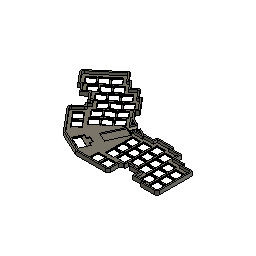
flynn (Autodesk Fusion 360 design; units mm, degrees)
Autodesk Fusion 360 part; units mm, degrees
(part 1 of 3)
sketch "Sketch1" plane through (0, 0, 0) normal (0, 1, 0) x (1, 0, 0)
  line L0 (0, 0) -> (0, -8) construction
  line L1 (0, -8) -> (8, -8) construction
  line L2 (8, -8) -> (22, -8)
  line L3 (22, -8) -> (22, -22)
  line L4 (22, -22) -> (8, -22)
  line L5 (8, -22) -> (8, -8)
  line L6 (8, -39) -> (8, -25)
  line L7 (8, -25) -> (22, -25)
  line L8 (22, -25) -> (22, -39)
  line L9 (22, -39) -> (8, -39)
  line L10 (8, -56) -> (8, -42)
  line L11 (8, -42) -> (22, -42)
  line L12 (22, -42) -> (22, -56)
  line L13 (22, -56) -> (8, -56)
  line L14 (22, -8) -> (22, -6) construction
  line L15 (22, -6) -> (26, -6) construction
  line L16 (26, -6) -> (40, -6)
  line L17 (40, -6) -> (40, -20)
  line L18 (40, -20) -> (26, -20)
  line L19 (26, -20) -> (26, -6)
  line L20 (26, -23) -> (40, -23)
  line L21 (40, -23) -> (40, -37)
  line L22 (40, -37) -> (26, -37)
  line L23 (26, -37) -> (26, -23)
  line L24 (26, -40) -> (40, -40)
  line L25 (40, -40) -> (40, -54)
  line L26 (40, -54) -> (26, -54)
  line L27 (26, -54) -> (26, -40)
  line L28 (40, -6) -> (40, 0) construction
  line L29 (40, 0) -> (44, 0) construction
  line L30 (44, 0) -> (58, 0)
  line L31 (58, 0) -> (58, -14)
  line L32 (58, -14) -> (44, -14)
  line L33 (44, -14) -> (44, 0)
  line L34 (58, -17) -> (58, -31)
  line L35 (44, -31) -> (44, -17)
  line L36 (58, -31) -> (44, -31)
  line L37 (44, -17) -> (58, -17)
  line L38 (58, -34) -> (58, -48)
  line L39 (44, -48) -> (44, -34)
  line L40 (58, -48) -> (44, -48)
  line L41 (44, -34) -> (58, -34)
  line L42 (58, 0) -> (62, 0) construction
  line L43 (62, 0) -> (62, -4) construction
  line L44 (62, -4) -> (76, -4)
  line L45 (76, -4) -> (76, -18)
  line L46 (76, -18) -> (62, -18)
  line L47 (62, -18) -> (62, -4)
  line L48 (76, -35) -> (62, -35)
  line L49 (62, -35) -> (62, -21)
  line L50 (76, -21) -> (76, -35)
  line L51 (62, -21) -> (76, -21)
  line L52 (76, -52) -> (62, -52)
  line L53 (62, -52) -> (62, -38)
  line L54 (76, -38) -> (76, -52)
  line L55 (62, -38) -> (76, -38)
  line L56 (76, -4) -> (80, -4) construction
  line L57 (80, -4) -> (80, -16) construction
  line L58 (80, -16) -> (94, -16)
  line L59 (94, -16) -> (94, -30)
  line L60 (94, -30) -> (80, -30)
  line L61 (80, -30) -> (80, -16)
  line L62 (94, -33) -> (94, -47)
  line L63 (80, -47) -> (80, -33)
  line L64 (94, -47) -> (80, -47)
  line L65 (80, -33) -> (94, -33)
  line L66 (94, -50) -> (94, -64)
  line L67 (80, -64) -> (80, -50)
  line L68 (94, -64) -> (80, -64)
  line L69 (80, -50) -> (94, -50)
  line L70 (94, -16) -> (98, -16) construction
  line L71 (98, -16) -> (98, -20) construction
  line L72 (98, -20) -> (112, -20)
  line L73 (112, -20) -> (112, -34)
  line L74 (112, -34) -> (98, -34)
  line L75 (98, -34) -> (98, -20)
  line L76 (98, -51) -> (98, -37)
  line L77 (112, -51) -> (98, -51)
  line L78 (112, -37) -> (112, -51)
  line L79 (98, -37) -> (112, -37)
  line L80 (98, -33) -> (98, -37) construction
  line L81 (98, -68) -> (98, -54)
  line L82 (112, -68) -> (98, -68)
  line L83 (112, -54) -> (112, -68)
  line L84 (98, -54) -> (112, -54)
  line L85 (98, -50) -> (98, -54) construction
  line L86 (22, -56) -> (22, -63) construction
  line L87 (22, -63) -> (19, -63) construction
  line L88 (19, -63) -> (33, -63)
  line L89 (33, -63) -> (33, -77)
  line L90 (33, -77) -> (19, -77)
  line L91 (19, -77) -> (19, -63)
  line L92 (15, -63) -> (15, -77)
  line L93 (1, -63) -> (15, -63)
  line L94 (4, -63) -> (1, -63) construction
  line L95 (15, -77) -> (1, -77)
  line L96 (1, -77) -> (1, -63)
  line L97 (26, -6) -> (26, 2) construction
  line L98 (26, 2) -> (18, 2) construction
  line L99 (40, 0) -> (48, 0) construction
  line L100 (44, 0) -> (44, 8) construction
  line L101 (44, 8) -> (36, 8) construction
  line L102 (58, 0) -> (58, 8) construction
  line L103 (58, 8) -> (66, 8) construction
  line L104 (62, -4) -> (62, 4) construction
  line L105 (62, 4) -> (70, 4) construction
  line L106 (76, -4) -> (76, 4) construction
  line L107 (76, 4) -> (84, 4) construction
  line L108 (80, -16) -> (80, -8) construction
  line L109 (80, -8) -> (88, -8) construction
  line L110 (94, -16) -> (94, -8) construction
  line L111 (94, -8) -> (102, -8) construction
  line L112 (98, -20) -> (98, -12) construction
  line L113 (98, -12) -> (106, -12) construction
  line L114 (112, -20) -> (112, -12) construction
  line L115 (112, -12) -> (120, -12) construction
  line L116 (0, 0) -> (18, 0)
  line L117 (18, 0) -> (18, 2)
  line L118 (18, 2) -> (36, 2)
  line L119 (36, 2) -> (36, 8)
  line L120 (36, 8) -> (61.9126, 8)
  line L121 (66, 8) -> (66, 4)
  line L122 (66, 4) -> (84, 4)
  line L123 (84, 4) -> (84, -8)
  line L124 (84, -8) -> (102, -8)
  line L125 (102, -8) -> (102, -12)
  line L126 (102, -12) -> (120, -12)
  line L127 (112, -68) -> (120, -68) construction
  line L128 (120, -68) -> (120, -76) construction
  line L129 (98, -68) -> (98, -76) construction
  line L130 (98, -76) -> (90, -76) construction
  line L131 (80, -64) -> (80, -72) construction
  line L132 (80, -72) -> (72, -72) construction
  line L133 (62, -52) -> (62, -60) construction
  line L134 (62, -60) -> (54, -60) construction
  line L135 (44, -48) -> (44, -56) construction
  line L136 (44, -56) -> (52, -56) construction
  line L137 (40, -54) -> (40, -62) construction
  line L138 (40, -62) -> (48, -62) construction
  line L139 (33, -63) -> (33, -55) construction
  line L140 (33, -55) -> (41, -55) construction
  line L141 (33, -77) -> (33, -85) construction
  line L142 (33, -85) -> (41, -85) construction
  line L143 (1, -77) -> (1, -85) construction
  line L144 (1, -85) -> (-7, -85) construction
  line L145 (1, -63) -> (1, -55) construction
  line L146 (1, -55) -> (-7, -55) construction
  line L147 (8, -56) -> (0, -56) construction
  line L148 (0, -56) -> (0, -48) construction
  line L149 (120, -12) -> (120, -76)
  line L150 (120, -76) -> (90, -76)
  line L151 (90, -76) -> (90, -72)
  line L152 (90, -72) -> (72, -72)
  line L153 (72, -72) -> (72, -60)
  line L154 (72, -60) -> (54, -60)
  line L155 (54, -60) -> (54, -56)
  line L156 (54, -56) -> (48, -56)
  line L157 (48, -56) -> (48, -62)
  line L158 (48, -62) -> (41, -62)
  line L159 (41, -62) -> (41, -85)
  line L160 (41, -85) -> (-7, -85)
  line L161 (-7, -85) -> (-7, -55)
  line L162 (-7, -55) -> (0, -55)
  line L163 (0, -55) -> (0, 0)
  line L164 (0, 0) -> (-4.5315, 2.1131)
  line L165 (-2.2658, 1.0565) -> (-5.5149, -5.9112)
  line L166 (-119.6157, 33.4759) -> (-108.8911, 42.4749)
  line L167 (-48.5486, -6.1026) -> (-39.5496, -16.8273)
  line L168 (-84.729, -22.1021) -> (-75.7299, -32.8267)
  line L169 (-14.5696, 17.1875) -> (-26.1398, 30.9763)
  line L170 (-65.0053, -23.8277) -> (-74.0043, -13.1031)
  line L171 (-19.7119, 23.3158) -> (-14.5696, 17.1875) construction
  line L172 (-95.9996, -21.116) -> (-65.1458, -57.8862)
  line L173 (-117.5376, 24.7764) -> (-105.9674, 10.9876)
  line L174 (-62.4342, -26.8919) -> (-73.1588, -35.8909)
  line L175 (-139.8854, 45.1866) -> (-120.6018, 22.2052)
  line L176 (-23.2691, 15.1093) -> (-25.8403, 18.1735) construction
  line L177 (-128.6148, 44.2005) -> (-133.7571, 50.3289) construction
  line L178 (-37.824, 2.8964) -> (-48.5486, -6.1026)
  line L179 (-82.4931, 35.9065) -> (-93.2177, 26.9075)
  line L180 (-105.9674, 10.9876) -> (-96.7749, 18.701)
  line L181 (-53.4351, -37.6165) -> (-62.4342, -26.8919)
  line L182 (-100.9577, 43.9103) -> (-91.9586, 33.1856)
  line L183 (-56.5616, 15.8926) -> (-45.8369, 24.8917)
  line L184 (-46.664, -33.2402) -> (-4.5315, 2.1131)
  line L185 (-55.3635, -35.3184) -> (-53.4351, -37.6165) construction
  line L186 (-71.1959, 27.1103) -> (-60.4713, 36.1093)
  line L187 (-125.7441, 28.3336) -> (-120.6018, 22.2052) construction
  line L188 (-69.4703, 46.8339) -> (-80.195, 37.8349)
  line L189 (-61.5714, -17.03) -> (-52.5723, -27.7547)
  line L190 (-108.8911, 42.4749) -> (-117.8902, 53.1995)
  line L191 (-104.9814, 22.2582) -> (-111.1097, 17.1159) construction
  line L192 (-91.8446, 75.0543) -> (-102.5693, 66.0553)
  line L193 (-77.2103, 63.8367) -> (-87.9349, 54.8376)
  line L194 (-47.43, -33.883) -> (-41.3017, -28.7407) construction
  line L195 (-93.5702, 55.3307) -> (-82.8456, 64.3297)
  line L196 (-50.8467, -8.031) -> (-61.5714, -17.03)
  line L197 (-94.2568, 31.2573) -> (-103.2558, 41.9819)
  line L198 (-64.1597, -46.6155) -> (-53.4351, -37.6165)
  line L199 (-42.1645, -38.6025) -> (-46.664, -33.2402)
  line L200 (-120.6018, 22.2052) -> (-117.5376, 24.7764)
  line L201 (-70.2881, -51.7578) -> (-65.1458, -57.8862) construction
  line L202 (-4.5315, 2.1131) -> (0, 0)
  line L203 (-102.5693, 66.0553) -> (-93.5702, 55.3307)
  line L204 (-55.4615, 69.032) -> (-64.6541, 61.3185)
  line L205 (-75.7299, -32.8267) -> (-65.0053, -23.8277)
  line L206 (-16.1017, 15.9019) -> (-14.5696, 17.1875)
  line L207 (-113.9804, 32.9829) -> (-104.9814, 22.2582)
  line L208 (-26.1398, 30.9763) -> (-21.5435, 34.833)
  line L209 (-24.8012, 13.8238) -> (-35.5258, 4.8247)
  line L210 (-115.592, 55.1279) -> (-106.593, 44.4033)
  line L211 (-76.7173, 69.472) -> (-81.8596, 75.6004) construction
  line L212 (-111.1097, 17.1159) -> (-105.9674, 10.9876) construction
  line L213 (-87.9349, 54.8376) -> (-78.9359, 44.113)
  line L214 (-56.4476, 57.7613) -> (-50.3192, 62.9036) construction
  line L215 (-56.4476, 57.7613) -> (-59.0187, 60.8255) construction
  line L216 (-74.0043, -13.1031) -> (-67.876, -7.9608) construction
  line L217 (-82.8456, 64.3297) -> (-76.7173, 69.472) construction
  line L218 (-56.4476, 57.7613) -> (-67.1722, 48.7623)
  line L219 (-76.2242, 75.1073) -> (-79.2884, 72.5362)
  line L220 (-91.9586, 33.1856) -> (-81.234, 42.1847)
  line L221 (-32.8142, 35.819) -> (-41.8132, 46.5437)
  line L222 (-81.234, 42.1847) -> (-90.233, 52.9093)
  line L223 (-25.8403, 18.1735) -> (-19.7119, 23.3158) construction
  line L224 (-61.5714, -17.03) -> (-66.9337, -21.5296) construction
  line L225 (-74.0043, -13.1031) -> (-84.729, -22.1021)
  line L226 (-90.233, 52.9093) -> (-100.9577, 43.9103)
  line L227 (-69.5843, 4.9652) -> (-75.7127, -0.1771) construction
  line L228 (-47.3068, -32.4742) -> (-42.1645, -38.6025) construction
  line L229 (-47.4485, 47.0367) -> (-41.3202, 52.179) construction
  line L230 (-59.0187, 60.8255) -> (-68.2113, 53.112) construction
  line L231 (-77.2103, 63.8367) -> (-79.7814, 66.9008) construction
  line L232 (-4.5315, 2.1131) -> (-10.6599, -3.0292) construction
  line L233 (-84.2187, 16.1829) -> (-73.4941, 25.1819)
  line L234 (-65.5606, 26.6173) -> (-56.5616, 15.8926)
  line L235 (-10.6599, -3.0292) -> (-15.8022, 3.0991) construction
  line L236 (-28.825, -7.8282) -> (-37.824, 2.8964)
  line L237 (-77.7378, -7.098) -> (-82.8801, -0.9696) construction
  line L238 (-49.5877, -1.7529) -> (-38.863, 7.2461)
  line L239 (-52.5723, -27.7547) -> (-41.8477, -18.7556)
  line L240 (-58.1732, 38.0377) -> (-47.4485, 47.0367)
  line L241 (-58.8597, 13.9643) -> (-67.8587, 24.6889)
  line L242 (-68.2113, 53.112) -> (-62.0829, 58.2543) construction
  line L243 (-92.8042, 55.9735) -> (-95.8684, 53.4023) construction
  line L244 (-43.8913, 55.2432) -> (-55.4615, 69.032)
  line L245 (-2.2658, 1.0565) -> (-5.5149, -5.9112)
  line L246 (-47.4485, 47.0367) -> (-56.4476, 57.7613)
  line L247 (-67.1722, 48.7623) -> (-58.1732, 38.0377)
  line L248 (-60.4713, 36.1093) -> (-69.4703, 46.8339)
  line L249 (-15.8022, 3.0991) -> (-24.8012, 13.8238)
  line L250 (-96.7749, 18.701) -> (-85.2047, 4.9122)
  line L251 (-85.7163, 80.1966) -> (-90.8586, 86.325) construction
  line L252 (-117.8902, 53.1995) -> (-128.6148, 44.2005)
  line L253 (-71.6094, -1.9557) -> (-77.7378, -7.098) construction
  line L254 (-105.8269, 45.0461) -> (-108.8911, 42.4749) construction
  line L255 (-60.8848, 7.0434) -> (-71.6094, -1.9557)
  line L256 (-84.729, -22.1021) -> (-90.8573, -27.2444) construction
  line L257 (-79.7814, 66.9008) -> (-82.8456, 64.3297) construction
  line L258 (-34.8393, 28.8981) -> (-30.243, 32.7549) construction
  line L259 (-78.2838, 2.8871) -> (-82.8801, -0.9696)
  line L260 (-79.2884, 72.5362) -> (-90.8586, 86.325)
  line L261 (-62.6104, -12.6803) -> (-51.8858, -3.6813)
  line L262 (-34.8393, 28.8981) -> (-45.5639, 19.8991)
  line L263 (-41.8132, 46.5437) -> (-44.3844, 49.6078) construction
  line L264 (-85.2047, 4.9122) -> (-82.1406, 7.4834)
  line L265 (-41.3202, 52.179) -> (-46.4625, 58.3074) construction
  line L266 (-64.6541, 61.3185) -> (-76.2242, 75.1073)
  line L267 (-69.5843, 4.9652) -> (-58.8597, 13.9643)
  line L268 (-82.8801, -0.9696) -> (-78.3806, -6.3319)
  line L269 (-47.8621, 17.9708) -> (-58.5867, 8.9717)
  line L270 (-30.243, 32.7549) -> (-35.3853, 38.8832) construction
  line L271 (-41.8132, 46.5437) -> (-52.5378, 37.5446)
  line L272 (-45.8369, 24.8917) -> (-54.836, 35.6163)
  line L273 (-35.6849, 51.686) -> (-40.8272, 57.8143) construction
  line L274 (-82.8456, 64.3297) -> (-91.8446, 75.0543)
  line L275 (-78.3806, -6.3319) -> (-95.9996, -21.116)
  line L276 (-58.5867, 8.9717) -> (-49.5877, -1.7529)
  line L277 (-71.6094, -1.9557) -> (-62.6104, -12.6803)
  line L278 (-77.2103, 63.8367) -> (-71.0819, 68.979) construction
  line L279 (-67.876, -7.9608) -> (-73.0183, -1.8324) construction
  line L280 (-32.8142, 35.819) -> (-26.6858, 40.9613) construction
  line L281 (-41.8132, 46.5437) -> (-35.6849, 51.686) construction
  line L282 (-40.8272, 57.8143) -> (-43.8913, 55.2432)
  line L283 (-91.8446, 75.0543) -> (-85.7163, 80.1966) construction
  line L284 (-75.7127, -0.1771) -> (-80.855, 5.9513) construction
  line L285 (-50.3192, 62.9036) -> (-55.4615, 69.032) construction
  line L286 (-78.5834, 15.6899) -> (-69.5843, 4.9652)
  line L287 (-84.2187, 16.1829) -> (-90.347, 11.0406) construction
  line L288 (-90.347, 11.0406) -> (-85.2047, 4.9122) construction
  line L289 (-45.5639, 19.8991) -> (-36.5649, 9.1745)
  line L290 (-43.5388, 26.82) -> (-32.8142, 35.819)
  line L291 (-38.863, 7.2461) -> (-47.8621, 17.9708)
  line L292 (-25.8403, 18.1735) -> (-34.8393, 28.8981)
  line L293 (-51.8858, -3.6813) -> (-60.8848, 7.0434)
  line L294 (-90.8573, -27.2444) -> (-95.9996, -21.116) construction
  line L295 (-82.1406, 7.4834) -> (-78.2838, 2.8871)
  line L296 (-26.6858, 40.9613) -> (-21.5435, 34.833) construction
  line L297 (-68.2113, 53.112) -> (-77.2103, 63.8367)
  line L298 (-71.0819, 68.979) -> (-76.2242, 75.1073) construction
  line L299 (-21.5435, 34.833) -> (-38.1998, 54.6832)
  line L300 (-67.8587, 24.6889) -> (-78.5834, 15.6899)
  line L301 (-30.243, 32.7549) -> (-32.8142, 35.819) construction
  line L302 (-44.3844, 49.6078) -> (-47.4485, 47.0367) construction
  line L303 (-52.5378, 37.5446) -> (-43.5388, 26.82)
  line L304 (-62.0829, 58.2543) -> (-67.2252, 64.3827) construction
  line L305 (-36.5649, 9.1745) -> (-25.8403, 18.1735)
  line L306 (-128.6148, 44.2005) -> (-119.6157, 33.4759)
  line L307 (-54.836, 35.6163) -> (-65.5606, 26.6173)
  line L308 (-104.9814, 22.2582) -> (-94.2568, 31.2573)
  line L309 (-90.8586, 86.325) -> (-139.8854, 45.1866)
  line L310 (-106.593, 44.4033) -> (-95.8684, 53.4023)
  line L311 (-52.5723, -27.7547) -> (-47.43, -33.883) construction
  line L312 (-95.8684, 53.4023) -> (-104.8674, 64.1269)
  line L313 (-39.5496, -16.8273) -> (-28.825, -7.8282)
  line L314 (-66.9337, -21.5296) -> (-65.0053, -23.8277) construction
  line L315 (-53.4351, -37.6165) -> (-47.3068, -32.4742) construction
  line L316 (-133.7571, 50.3289) -> (-139.8854, 45.1866) construction
  line L317 (-78.9359, 44.113) -> (-68.2113, 53.112)
  line L318 (-64.1597, -46.6155) -> (-70.2881, -51.7578) construction
  line L319 (-80.195, 37.8349) -> (-71.1959, 27.1103)
  line L320 (-4.5315, 2.1131) -> (-16.1017, 15.9019)
  line L321 (-65.1458, -57.8862) -> (-42.1645, -38.6025)
  line L322 (-103.2558, 41.9819) -> (-113.9804, 32.9829)
  line L323 (-73.1588, -35.8909) -> (-64.1597, -46.6155)
  line L324 (-93.2177, 26.9075) -> (-84.2187, 16.1829)
  line L325 (-73.4941, 25.1819) -> (-82.4931, 35.9065)
  line L326 (-41.8477, -18.7556) -> (-50.8467, -8.031)
  line L327 (-24.8012, 13.8238) -> (-23.2691, 15.1093) construction
  line L328 (-104.8674, 64.1269) -> (-115.592, 55.1279)
  line L329 (-119.6157, 33.4759) -> (-125.7441, 28.3336) construction
  line L330 (-26.5268, -5.8999) -> (-15.8022, 3.0991)
  line L331 (-35.5258, 4.8247) -> (-26.5268, -5.8999)
  line L332 (-7, -85) -> (-17, -85)
  line L333 (-65.1458, -57.8862) -> (-58.7179, -65.5466)
  line L334 (-58.7179, -65.5466) -> (-17, -85)
  line L335 (61.9126, 8) -> (66, 8)
  line L336 (-40.8272, 57.8143) -> (-35.6849, 51.686)
  point P0 (-4.5315, 2.1131)
  dimension "d1" = 8
  dimension "d3" = 14
  dimension "d4" = 14
  dimension "d7" = 0
  dimension "d8" = -17
  dimension "d9" = 2
  dimension "d10" = 4
  dimension "d11" = 14
  dimension "d12" = 14
  dimension "d15" = 0
  dimension "d16" = -17
  dimension "d17" = 14
  dimension "d18" = 14
  dimension "d19" = 4
  dimension "d20" = 6
  dimension "d23" = 0
  dimension "d24" = -17
  dimension "d25" = 4
  dimension "d26" = 4
  dimension "d27" = 14
  dimension "d28" = 14
  dimension "d31" = 0
  dimension "d32" = -17
  dimension "d33" = 12
  dimension "d34" = 4
  dimension "d35" = 14
  dimension "d36" = 14
  dimension "d39" = 0
  dimension "d40" = -17
  dimension "d41" = 4
  dimension "d42" = 4
  dimension "d43" = 14
  dimension "d44" = 14
  dimension "d47" = 0
  dimension "d48" = -17
  dimension "d49" = 14
  dimension "d50" = 14
  dimension "d51" = 7
  dimension "d52" = 3
  dimension "d55" = -18
  dimension "d56" = 0
  dimension "d57" = 5
  dimension "d58" = 155
  dimension "d68" = 10
  constraint coincident L0.start L116.start
  constraint vertical L0
  constraint perpendicular L0 L1
  constraint horizontal L2
  constraint vertical L3
  constraint horizontal L4
  constraint vertical L5
  constraint perpendicular L2 L14
  constraint perpendicular L14 L15
  constraint horizontal L16
  constraint vertical L17
  constraint horizontal L18
  constraint vertical L19
  constraint perpendicular L16 L28
  constraint perpendicular L28 L29
  constraint horizontal L30
  constraint vertical L31
  constraint horizontal L32
  constraint vertical L33
  constraint perpendicular L31 L42
  constraint perpendicular L30 L43
  constraint horizontal L44
  constraint vertical L45
  constraint horizontal L46
  constraint vertical L47
  constraint perpendicular L45 L56
  constraint perpendicular L56 L57
  constraint horizontal L58
  constraint vertical L59
  constraint horizontal L60
  constraint vertical L61
  constraint perpendicular L59 L70
  constraint perpendicular L58 L71
  constraint horizontal L72
  constraint vertical L73
  constraint horizontal L74
  constraint vertical L75
  constraint perpendicular L13 L86
  constraint perpendicular L86 L87
  constraint horizontal L88
  constraint vertical L89
  constraint horizontal L90
  constraint vertical L91
  constraint equal L0 L1
  constraint perpendicular L16 L97
  constraint perpendicular L19 L98
  constraint equal L0 L97
  constraint equal L0 L98
  constraint coincident L30 L99.end
  constraint equal L0 L99
  constraint perpendicular L99 L100
  constraint perpendicular L100 L101
  constraint equal L0 L100
  constraint equal L0 L101
  constraint perpendicular L30 L102
  constraint perpendicular L102 L103
  constraint equal L0 L102
  constraint equal L0 L103
  constraint perpendicular L44 L104
  constraint perpendicular L104 L105
  constraint equal L103 L105
  constraint equal L102 L104
  constraint perpendicular L56 L106
  constraint perpendicular L106 L107
  constraint equal L0 L107
  constraint equal L0 L106
  constraint coincident L57 L108.end
  constraint perpendicular L58 L108
  constraint perpendicular L108 L109
  constraint equal L0 L109
  constraint equal L0 L108
  constraint perpendicular L70 L110
  constraint perpendicular L59 L111
  constraint equal L0 L111
  constraint equal L0 L110
  constraint perpendicular L70 L112
  constraint perpendicular L112 L113
  constraint equal L0 L113
  constraint equal L0 L112
  constraint perpendicular L72 L114
  constraint perpendicular L114 L115
  constraint equal L0 L115
  constraint equal L0 L114
  constraint perpendicular L97 L116
  constraint perpendicular L98 L117
  constraint perpendicular L117 L118
  constraint perpendicular L101 L119
  constraint perpendicular L119 L120
  constraint coincident L105 L121.end
  constraint perpendicular L105 L121
  constraint coincident L109 L123.end
  constraint perpendicular L109 L123
  constraint coincident L113 L125.end
  constraint perpendicular L113 L125
  constraint perpendicular L83 L127
  constraint perpendicular L82 L128
  constraint equal L0 L127
  constraint equal L0 L128
  constraint perpendicular L82 L129
  constraint perpendicular L129 L130
  constraint equal L0 L129
  constraint equal L0 L130
  constraint perpendicular L68 L131
  constraint perpendicular L131 L132
  constraint equal L0 L131
  constraint equal L0 L132
  constraint perpendicular L52 L133
  constraint perpendicular L53 L134
  constraint equal L0 L133
  constraint equal L0 L134
  constraint perpendicular L40 L135
  constraint perpendicular L135 L136
  constraint equal L0 L135
  constraint equal L0 L136
  constraint perpendicular L26 L137
  constraint perpendicular L137 L138
  constraint equal L0 L137
  constraint equal L0 L138
  constraint perpendicular L88 L139
  constraint perpendicular L139 L140
  constraint equal L0 L140
  constraint equal L0 L139
  constraint perpendicular L90 L141
  constraint perpendicular L141 L142
  constraint equal L0 L141
  constraint equal L0 L142
  constraint perpendicular L95 L143
  constraint perpendicular L143 L144
  constraint equal L0 L143
  constraint equal L0 L144
  constraint perpendicular L93 L145
  constraint perpendicular L96 L146
  constraint equal L0 L145
  constraint equal L0 L146
  constraint perpendicular L10 L147
  constraint perpendicular L13 L148
  constraint equal L0 L148
  constraint equal L0 L147
  constraint perpendicular L132 L151
  constraint perpendicular L131 L152
  constraint perpendicular L134 L153
  constraint perpendicular L133 L154
  constraint perpendicular L136 L155
  constraint coincident L136 L156.end
  constraint perpendicular L155 L156
  constraint perpendicular L138 L157
  constraint perpendicular L137 L158
  constraint perpendicular L142 L159
  constraint perpendicular L148 L162
  constraint perpendicular L116 L163
  constraint midpoint L164 L165.start
  constraint perpendicular L164 L165
  constraint symmetric L0.start L165 L164.end
  constraint symmetric L0.start L165 P0
  constraint symmetric L0.end L165 L232.end
  constraint symmetric L1.end L165 L235.end
  constraint symmetric L2.end L165 L209.start
  constraint symmetric L3.end L165 L209.end
  constraint symmetric L4.end L165 L330.start
  constraint symmetric L6.start L165 L167.end
  constraint symmetric L6.end L165 L236.start
  constraint symmetric L7.end L165 L178.start
  constraint symmetric L8.end L165 L167.start
  constraint symmetric L10.start L165 L189.end
  constraint symmetric L10.end L165 L239.end
  constraint symmetric L11.end L165 L196.start
  constraint symmetric L12.end L165 L189.start
  constraint symmetric L14.end L165 L176.start
  constraint symmetric L15.end L165 L176.end
  constraint symmetric L16.end L165 L258.start
  constraint symmetric L17.end L165 L262.end
  constraint symmetric L18.end L165 L289.end
  constraint symmetric L21.end L165 L269.end
  constraint symmetric L20.start L165 L238.end
  constraint symmetric L20.end L165 L269.start
  constraint symmetric L22.end L165 L238.start
  constraint symmetric L25.end L165 L253.start
  constraint symmetric L24.start L165 L261.end
  constraint symmetric L24.end L165 L255.start
  constraint symmetric L26.end L165 L261.start
  constraint symmetric L28.end L165 L258.end
  constraint symmetric L29.end L165 L221.start
  constraint symmetric L30.end L165 L221.end
  constraint symmetric L31.end L165 L271.end
  constraint symmetric L32.end L165 L290.start
  constraint symmetric L34.start L165 L272.end
  constraint symmetric L34.end L165 L234.start
  constraint symmetric L35.start L165 L183.start
  constraint symmetric L35.end L165 L183.end
  constraint symmetric L38.start L165 L241.end
  constraint symmetric L38.end L165 L286.start
  constraint symmetric L39.start L165 L227.start
  constraint symmetric L39.end L165 L241.start
  constraint symmetric L42.end L165 L263.end
  constraint symmetric L43.end L165 L229.start
  constraint symmetric L44.end L165 L214.start
  constraint symmetric L45.end L165 L218.end
  constraint symmetric L46.end L165 L240.start
  constraint symmetric L48.start L165 L188.end
  constraint symmetric L48.end L165 L186.start
  constraint symmetric L49.end L165 L186.end
  constraint symmetric L50.start L165 L188.start
  constraint symmetric L52.start L165 L179.end
  constraint symmetric L52.end L165 L233.start
  constraint symmetric L53.end L165 L233.end
  constraint symmetric L54.start L165 L179.start
  constraint symmetric L56.end L165 L215.end
  constraint symmetric L57.end L165 L230.end
  constraint symmetric L58.end L165 L193.start
  constraint symmetric L59.end L165 L193.end
  constraint symmetric L60.end L165 L213.end
  constraint symmetric L63.end L165 L220.end
  constraint symmetric L62.start L165 L222.end
  constraint symmetric L62.end L165 L182.start
  constraint symmetric L63.start L165 L182.end
  constraint symmetric L67.end L165 L197.start
  constraint symmetric L66.start L165 L197.end
  constraint symmetric L66.end L165 L207.start
  constraint symmetric L67.start L165 L191.start
  constraint symmetric L70.end L165 L231.end
  constraint symmetric L71.end L165 L195.end
  constraint symmetric L72.end L165 L192.start
  constraint symmetric L73.end L165 L192.end
  constraint symmetric L74.end L165 L195.start
  constraint symmetric L76.start L165 L210.end
  constraint symmetric L76.end L165 L243.end
  constraint symmetric L77.start L165 L210.start
  constraint symmetric L78.start L165 L312.end
  constraint symmetric L80.start L165 L243.start
  constraint symmetric L81.start L165 L166.start
  constraint symmetric L81.end L165 L166.end
  constraint symmetric L82.start L165 L177.start
  constraint symmetric L83.start L165 L190.end
  constraint symmetric L85.start L165 L254.start
  constraint symmetric L86.end L165 L224.end
  constraint symmetric L87.end L165 L170.start
  constraint symmetric L88.end L165 L170.end
  constraint symmetric L89.end L165 L168.start
  constraint symmetric L90.end L165 L168.end
  constraint symmetric L95.end L165 L198.start
  constraint symmetric L92.start L165 L174.start
  constraint symmetric L92.end L165 L174.end
  constraint symmetric L93.start L165 L181.start
  constraint symmetric L94.start L165 L185.start
  constraint symmetric L97.end L165 L171.start
  constraint symmetric L98.end L165 L169.start
  constraint symmetric L99.end L165 L270.end
  constraint symmetric L100.end L165 L280.end
  constraint symmetric L101.end L165 L208.end
  constraint symmetric L102.end L165 L273.start
  constraint symmetric L103.end L165 L273.end
  constraint symmetric L104.end L165 L229.end
  constraint symmetric L105.end L165 L265.end
  constraint symmetric L106.end L165 L214.end
  constraint symmetric L107.end L165 L204.start
  constraint symmetric L108.end L165 L242.end
  constraint symmetric L109.end L165 L304.end
  constraint symmetric L110.end L165 L278.end
  constraint symmetric L111.end L165 L219.start
  constraint symmetric L112.end L165 L211.start
  constraint symmetric L113.end L165 L211.end
  constraint symmetric L114.end L165 L251.start
  constraint symmetric L115.end L165 L251.end
  constraint symmetric L116.end L165 L206.start
  constraint symmetric L118.end L165 L169.end
  constraint symmetric L120.end L165 L299.end
  constraint symmetric L121.end L165 L244.start
  constraint symmetric L123.end L165 L204.end
  constraint symmetric L125.end L165 L219.end
  constraint symmetric L127.end L165 L177.end
  constraint symmetric L128.end L165 L175.start
  constraint symmetric L129.end L165 L187.start
  constraint symmetric L130.end L165 L175.end
  constraint symmetric L131.end L165 L191.end
  constraint symmetric L132.end L165 L173.end
  constraint symmetric L133.end L165 L287.end
  constraint symmetric L134.end L165 L250.end
  constraint symmetric L135.end L165 L227.end
  constraint symmetric L136.end L165 L284.end
  constraint symmetric L137.end L165 L237.start
  constraint symmetric L138.end L165 L237.end
  constraint symmetric L139.end L165 L216.end
  constraint symmetric L140.end L165 L279.end
  constraint symmetric L141.end L165 L256.end
  constraint symmetric L142.end L165 L172.start
  constraint symmetric L143.end L165 L201.start
  constraint symmetric L144.end L165 L172.end
  constraint symmetric L145.end L165 L228.start
  constraint symmetric L146.end L165 L199.start
  constraint symmetric L147.end L165 L194.start
  constraint symmetric L148.end L165 L194.end
  constraint symmetric L151.end L165 L173.start
  constraint symmetric L153.end L165 L180.end
  constraint symmetric L155.end L165 L264.end
  constraint symmetric L156.end L165 L259.start
  constraint symmetric L158.end L165 L268.end
  constraint symmetric L162.end L165 L184.start
  constraint symmetric P0 L165 L0.start
  constraint symmetric L245.start L165 L165.start
  constraint symmetric L245.end L165 L165.end
  constraint perpendicular L161 L332
  constraint perpendicular L321 L333
  constraint equal L332 L333
  constraint perpendicular L121 L335
  measures "d1" distance of L0.start L0.end
  measures "d3" distance of L1.end L2.end
  measures "d4" distance of L1.end L4.end
  measures "d9" distance of L2.end L14.end
  measures "d10" distance of L14.end L15.end
  measures "d11" distance of L15.end L16.end
  measures "d12" distance of L15.end L18.end
  measures "d17" distance of L29.end L30.end
  measures "d18" distance of L29.end L32.end
  measures "d19" distance of L28.end L29.end
  measures "d20" distance of L16.end L28.end
  measures "d25" distance of L30.end L42.end
  measures "d26" distance of L42.end L43.end
  measures "d27" distance of L43.end L44.end
  measures "d28" distance of L43.end L46.end
  measures "d33" distance of L56.end L57.end
  measures "d34" distance of L44.end L56.end
  measures "d35" distance of L57.end L58.end
  measures "d36" distance of L57.end L60.end
  measures "d41" distance of L58.end L70.end
  measures "d42" distance of L70.end L71.end
  measures "d43" distance of L71.end L72.end
  measures "d44" distance of L71.end L74.end
  measures "d49" distance of L87.end L88.end
  measures "d50" distance of L87.end L90.end
  measures "d51" distance of L12.end L86.end
  measures "d52" distance of L86.end L87.end
  measures "d57" distance of L0.start P0
  measures "d58" angle of L116 L164
  measures "d68" distance of L172.end L333.end
extrude "Extrude1" add sketch "Sketch1" along normal blind 1.3
sketch "Sketch15" plane through (0, 1.3, 0) normal (0, 1, 0) x (-1, 0, 0)
  line L0 (91.8446, -75.0543) -> (82.8456, -64.3297)
  line L1 (82.8456, -64.3297) -> (93.5702, -55.3307)
  line L2 (93.5702, -55.3307) -> (102.5693, -66.0553)
  line L3 (102.5693, -66.0553) -> (91.8446, -75.0543)
  line L4 (100.9577, -43.9103) -> (90.233, -52.9093)
  line L5 (90.233, -52.9093) -> (81.234, -42.1847)
  line L6 (81.234, -42.1847) -> (91.9586, -33.1856)
  line L7 (91.9586, -33.1856) -> (100.9577, -43.9103)
  line L8 (58.1732, -38.0377) -> (67.1722, -48.7623)
  line L9 (67.1722, -48.7623) -> (56.4476, -57.7613)
  line L10 (56.4476, -57.7613) -> (47.4485, -47.0367)
  line L11 (47.4485, -47.0367) -> (58.1732, -38.0377)
  line L12 (43.5388, -26.82) -> (52.5378, -37.5446)
  line L13 (52.5378, -37.5446) -> (41.8132, -46.5437)
  line L14 (41.8132, -46.5437) -> (32.8142, -35.819)
  line L15 (32.8142, -35.819) -> (43.5388, -26.82)
  line L16 (78.5834, -15.6899) -> (67.8587, -24.6889)
  line L17 (67.8587, -24.6889) -> (58.8597, -13.9643)
  line L18 (58.8597, -13.9643) -> (69.5843, -4.9652)
  line L19 (69.5843, -4.9652) -> (78.5834, -15.6899)
  line L20 (60.8848, -7.0434) -> (51.8858, 3.6813)
  line L21 (51.8858, 3.6813) -> (62.6104, 12.6803)
  line L22 (62.6104, 12.6803) -> (71.6094, 1.9557)
  line L23 (71.6094, 1.9557) -> (60.8848, -7.0434)
  line L24 (47.8621, -17.9708) -> (38.863, -7.2461)
  line L25 (38.863, -7.2461) -> (49.5877, 1.7529)
  line L26 (49.5877, 1.7529) -> (58.5867, -8.9717)
  line L27 (58.5867, -8.9717) -> (47.8621, -17.9708)
  line L28 (25.8403, -18.1735) -> (36.5649, -9.1745)
  line L29 (36.5649, -9.1745) -> (45.5639, -19.8991)
  line L30 (45.5639, -19.8991) -> (34.8393, -28.8981)
  line L31 (34.8393, -28.8981) -> (25.8403, -18.1735)
  line L32 (119.6157, -33.4759) -> (128.6148, -44.2005)
  line L33 (128.6148, -44.2005) -> (117.8902, -53.1995)
  line L34 (117.8902, -53.1995) -> (108.8911, -42.4749)
  line L35 (108.8911, -42.4749) -> (119.6157, -33.4759)
  line L36 (65.5606, -26.6173) -> (54.836, -35.6163)
  line L37 (54.836, -35.6163) -> (45.8369, -24.8917)
  line L38 (45.8369, -24.8917) -> (56.5616, -15.8926)
  line L39 (56.5616, -15.8926) -> (65.5606, -26.6173)
  line L40 (28.825, 7.8282) -> (39.5496, 16.8273)
  line L41 (39.5496, 16.8273) -> (48.5486, 6.1026)
  line L42 (48.5486, 6.1026) -> (37.824, -2.8964)
  line L43 (37.824, -2.8964) -> (28.825, 7.8282)
  line L44 (68.2113, -53.112) -> (78.9359, -44.113)
  line L45 (78.9359, -44.113) -> (87.9349, -54.8376)
  line L46 (87.9349, -54.8376) -> (77.2103, -63.8367)
  line L47 (77.2103, -63.8367) -> (68.2113, -53.112)
  line L48 (71.1959, -27.1103) -> (80.195, -37.8349)
  line L49 (80.195, -37.8349) -> (69.4703, -46.8339)
  line L50 (69.4703, -46.8339) -> (60.4713, -36.1093)
  line L51 (60.4713, -36.1093) -> (71.1959, -27.1103)
  line L52 (113.9804, -32.9829) -> (103.2558, -41.9819)
  line L53 (103.2558, -41.9819) -> (94.2568, -31.2573)
  line L54 (94.2568, -31.2573) -> (104.9814, -22.2582)
  line L55 (104.9814, -22.2582) -> (113.9804, -32.9829)
  line L56 (64.1597, 46.6155) -> (73.1588, 35.8909)
  line L57 (73.1588, 35.8909) -> (62.4342, 26.8919)
  line L58 (62.4342, 26.8919) -> (53.4351, 37.6165)
  line L59 (53.4351, 37.6165) -> (64.1597, 46.6155)
  line L60 (82.4931, -35.9065) -> (73.4941, -25.1819)
  line L61 (73.4941, -25.1819) -> (84.2187, -16.1829)
  line L62 (84.2187, -16.1829) -> (93.2177, -26.9075)
  line L63 (93.2177, -26.9075) -> (82.4931, -35.9065)
  line L64 (50.8467, 8.031) -> (41.8477, 18.7556)
  line L65 (41.8477, 18.7556) -> (52.5723, 27.7547)
  line L66 (52.5723, 27.7547) -> (61.5714, 17.03)
  line L67 (61.5714, 17.03) -> (50.8467, 8.031)
  line L68 (115.592, -55.1279) -> (104.8674, -64.1269)
  line L69 (104.8674, -64.1269) -> (95.8684, -53.4023)
  line L70 (95.8684, -53.4023) -> (106.593, -44.4033)
  line L71 (106.593, -44.4033) -> (115.592, -55.1279)
  line L72 (-15, 77) -> (-1, 77)
  line L73 (-1, 77) -> (-1, 63)
  line L74 (-1, 63) -> (-15, 63)
  line L75 (-15, 63) -> (-15, 77)
  line L76 (84.729, 22.1021) -> (74.0043, 13.1031)
  line L77 (74.0043, 13.1031) -> (65.0053, 23.8277)
  line L78 (65.0053, 23.8277) -> (75.7299, 32.8267)
  line L79 (75.7299, 32.8267) -> (84.729, 22.1021)
  line L80 (-33, 77) -> (-19, 77)
  line L81 (-19, 77) -> (-19, 63)
  line L82 (-19, 63) -> (-33, 63)
  line L83 (-33, 63) -> (-33, 77)
  line L84 (-98, 68) -> (-98, 54)
  line L85 (-98, 54) -> (-112, 54)
  line L86 (-112, 54) -> (-112, 68)
  line L87 (-112, 68) -> (-98, 68)
  line L88 (-98, 51) -> (-98, 37)
  line L89 (-98, 37) -> (-112, 37)
  line L90 (-112, 37) -> (-112, 51)
  line L91 (-112, 51) -> (-98, 51)
  line L92 (-62, 52) -> (-62, 38)
  line L93 (-62, 38) -> (-76, 38)
  line L94 (-76, 38) -> (-76, 52)
  line L95 (-76, 52) -> (-62, 52)
  line L96 (-112, 34) -> (-98, 34)
  line L97 (-98, 34) -> (-98, 20)
  line L98 (-98, 20) -> (-112, 20)
  line L99 (-112, 20) -> (-112, 34)
  line L100 (-94, 30) -> (-80, 30)
  line L101 (-80, 30) -> (-80, 16)
  line L102 (-80, 16) -> (-94, 16)
  line L103 (-94, 16) -> (-94, 30)
  line L104 (-80, 64) -> (-80, 50)
  line L105 (-80, 50) -> (-94, 50)
  line L106 (-94, 50) -> (-94, 64)
  line L107 (-94, 64) -> (-80, 64)
  line L108 (-80, 47) -> (-80, 33)
  line L109 (-80, 33) -> (-94, 33)
  line L110 (-94, 33) -> (-94, 47)
  line L111 (-94, 47) -> (-80, 47)
  line L112 (-62, 35) -> (-62, 21)
  line L113 (-62, 21) -> (-76, 21)
  line L114 (-76, 21) -> (-76, 35)
  line L115 (-76, 35) -> (-62, 35)
  line L116 (-76, 18) -> (-62, 18)
  line L117 (-62, 18) -> (-62, 4)
  line L118 (-62, 4) -> (-76, 4)
  line L119 (-76, 4) -> (-76, 18)
  line L120 (-44, 48) -> (-44, 34)
  line L121 (-44, 34) -> (-58, 34)
  line L122 (-58, 34) -> (-58, 48)
  line L123 (-58, 48) -> (-44, 48)
  line L124 (-44, 31) -> (-44, 17)
  line L125 (-44, 17) -> (-58, 17)
  line L126 (-58, 17) -> (-58, 31)
  line L127 (-58, 31) -> (-44, 31)
  line L128 (-58, 14) -> (-44, 14)
  line L129 (-44, 14) -> (-44, 0)
  line L130 (-44, 0) -> (-58, 0)
  line L131 (-58, 0) -> (-58, 14)
  line L132 (-40, 54) -> (-26, 54)
  line L133 (-26, 54) -> (-26, 40)
  line L134 (-26, 40) -> (-40, 40)
  line L135 (-40, 40) -> (-40, 54)
  line L136 (-40, 37) -> (-26, 37)
  line L137 (-26, 37) -> (-26, 23)
  line L138 (-26, 23) -> (-40, 23)
  line L139 (-40, 23) -> (-40, 37)
  line L140 (-40, 20) -> (-26, 20)
  line L141 (-26, 20) -> (-26, 6)
  line L142 (-26, 6) -> (-40, 6)
  line L143 (-40, 6) -> (-40, 20)
  line L144 (-22, 42) -> (-22, 56)
  line L145 (-22, 56) -> (-8, 56)
  line L146 (-8, 56) -> (-8, 42)
  line L147 (-8, 42) -> (-22, 42)
  line L148 (-22, 25) -> (-22, 39)
  line L149 (-22, 39) -> (-8, 39)
  line L150 (-8, 39) -> (-8, 25)
  line L151 (-8, 25) -> (-22, 25)
  line L152 (-22, 22) -> (-8, 22)
  line L153 (-8, 22) -> (-8, 8)
  line L154 (-8, 8) -> (-22, 8)
  line L155 (-22, 8) -> (-22, 22)
  line L156 (26.5268, 5.8999) -> (35.5258, -4.8247)
  line L157 (35.5258, -4.8247) -> (24.8012, -13.8238)
  line L158 (24.8012, -13.8238) -> (15.8022, -3.0991)
  line L159 (15.8022, -3.0991) -> (26.5268, 5.8999)
  line L160 (43.8913, -55.2432) -> (55.4615, -69.032)
  line L161 (55.4615, -69.032) -> (64.6541, -61.3185)
  line L162 (64.6541, -61.3185) -> (76.2242, -75.1073)
  line L163 (76.2242, -75.1073) -> (79.2884, -72.5362)
  line L164 (79.2884, -72.5362) -> (90.8586, -86.325)
  line L165 (90.8586, -86.325) -> (139.8854, -45.1866)
  line L166 (139.8854, -45.1866) -> (120.6018, -22.2052)
  line L167 (120.6018, -22.2052) -> (117.5376, -24.7764)
  line L168 (117.5376, -24.7764) -> (105.9674, -10.9876)
  line L169 (105.9674, -10.9876) -> (96.7749, -18.701)
  line L170 (96.7749, -18.701) -> (85.2047, -4.9122)
  line L171 (85.2047, -4.9122) -> (82.1406, -7.4834)
  line L172 (82.1406, -7.4834) -> (78.2838, -2.8871)
  line L173 (78.2838, -2.8871) -> (82.8801, 0.9696)
  line L174 (82.8801, 0.9696) -> (78.3806, 6.3319)
  line L175 (78.3806, 6.3319) -> (95.9996, 21.116)
  line L176 (95.9996, 21.116) -> (58.7179, 65.5466)
  line L177 (58.7179, 65.5466) -> (17, 85)
  line L178 (17, 85) -> (-41, 85)
  line L179 (-41, 85) -> (-41, 62)
  line L180 (-41, 62) -> (-48, 62)
  line L181 (-48, 62) -> (-48, 56)
  line L182 (-48, 56) -> (-54, 56)
  line L183 (-54, 56) -> (-54, 60)
  line L184 (-54, 60) -> (-72, 60)
  line L185 (-72, 60) -> (-72, 72)
  line L186 (-72, 72) -> (-90, 72)
  line L187 (-90, 72) -> (-90, 76)
  line L188 (-90, 76) -> (-120, 76)
  line L189 (-120, 76) -> (-120, 12)
  line L190 (-120, 12) -> (-102, 12)
  line L191 (-102, 12) -> (-102, 8)
  line L192 (-102, 8) -> (-84, 8)
  line L193 (-84, 8) -> (-84, -4)
  line L194 (-84, -4) -> (-66, -4)
  line L195 (-66, -4) -> (-66, -8)
  line L196 (-66, -8) -> (-36, -8)
  line L197 (-36, -8) -> (-36, -2)
  line L198 (-36, -2) -> (-18, -2)
  line L199 (-18, -2) -> (-18, 0)
  line L200 (-18, 0) -> (0, 0)
  line L201 (0, 0) -> (4.5315, -2.1131)
  line L202 (4.5315, -2.1131) -> (16.1017, -15.9019)
  line L203 (16.1017, -15.9019) -> (14.5696, -17.1875)
  line L204 (14.5696, -17.1875) -> (26.1398, -30.9763)
  line L205 (26.1398, -30.9763) -> (21.5435, -34.833)
  line L206 (21.5435, -34.833) -> (40.8272, -57.8143)
  line L207 (40.8272, -57.8143) -> (43.8913, -55.2432)
  line L208 (-7.5, 24.5) -> (-22.5, 24.5)
  line L209 (-22.5, 24.5) -> (-22.5, 39.5)
  line L210 (-22.5, 39.5) -> (-7.5, 39.5)
  line L211 (-7.5, 39.5) -> (-7.5, 24.5)
  line L212 (-0.5, 77.5) -> (-0.5, 62.5)
  line L213 (-0.5, 62.5) -> (-15.5, 62.5)
  line L214 (-15.5, 62.5) -> (-15.5, 77.5)
  line L215 (-15.5, 77.5) -> (-0.5, 77.5)
  line L216 (117.8285, -53.904) -> (108.1867, -42.4133)
  line L217 (108.1867, -42.4133) -> (119.6774, -32.7715)
  line L218 (119.6774, -32.7715) -> (129.3192, -44.2621)
  line L219 (129.3192, -44.2621) -> (117.8285, -53.904)
  line L220 (90.1714, -53.6137) -> (80.5296, -42.123)
  line L221 (80.5296, -42.123) -> (92.0203, -32.4812)
  line L222 (92.0203, -32.4812) -> (101.6621, -43.9719)
  line L223 (101.6621, -43.9719) -> (90.1714, -53.6137)
  line L224 (53.2423, -37.6063) -> (41.7516, -47.2481)
  line L225 (41.7516, -47.2481) -> (32.1098, -35.7574)
  line L226 (32.1098, -35.7574) -> (43.6004, -26.1156)
  line L227 (43.6004, -26.1156) -> (53.2423, -37.6063)
  line L228 (37.7623, -3.6008) -> (28.1205, 7.8899)
  line L229 (28.1205, 7.8899) -> (39.6112, 17.5317)
  line L230 (39.6112, 17.5317) -> (49.253, 6.041)
  line L231 (49.253, 6.041) -> (37.7623, -3.6008)
  line L232 (-97.5, 36.5) -> (-112.5, 36.5)
  line L233 (-112.5, 36.5) -> (-112.5, 51.5)
  line L234 (-112.5, 51.5) -> (-97.5, 51.5)
  line L235 (-97.5, 51.5) -> (-97.5, 36.5)
  line L236 (-25.5, 22.5) -> (-40.5, 22.5)
  line L237 (-40.5, 22.5) -> (-40.5, 37.5)
  line L238 (-40.5, 37.5) -> (-25.5, 37.5)
  line L239 (-25.5, 37.5) -> (-25.5, 22.5)
  line L240 (78.9975, -43.4086) -> (88.6393, -54.8993)
  line L241 (88.6393, -54.8993) -> (77.1487, -64.5411)
  line L242 (77.1487, -64.5411) -> (67.5068, -53.0504)
  line L243 (67.5068, -53.0504) -> (78.9975, -43.4086)
  line L244 (-43.5, 48.5) -> (-43.5, 33.5)
  line L245 (-43.5, 33.5) -> (-58.5, 33.5)
  line L246 (-58.5, 33.5) -> (-58.5, 48.5)
  line L247 (-58.5, 48.5) -> (-43.5, 48.5)
  line L248 (52.7307, 37.6781) -> (64.2214, 47.3199)
  line L249 (64.2214, 47.3199) -> (73.8632, 35.8293)
  line L250 (73.8632, 35.8293) -> (62.3725, 26.1874)
  line L251 (62.3725, 26.1874) -> (52.7307, 37.6781)
  line L252 (46.2683, -19.9607) -> (34.7777, -29.6026)
  line L253 (34.7777, -29.6026) -> (25.1359, -18.1119)
  line L254 (25.1359, -18.1119) -> (36.6265, -8.4701)
  line L255 (36.6265, -8.4701) -> (46.2683, -19.9607)
  line L256 (-25.5, 20.5) -> (-25.5, 5.5)
  line L257 (-25.5, 5.5) -> (-40.5, 5.5)
  line L258 (-40.5, 5.5) -> (-40.5, 20.5)
  line L259 (-40.5, 20.5) -> (-25.5, 20.5)
  line L260 (-61.5, 3.5) -> (-76.5, 3.5)
  line L261 (-76.5, 3.5) -> (-76.5, 18.5)
  line L262 (-76.5, 18.5) -> (-61.5, 18.5)
  line L263 (-61.5, 18.5) -> (-61.5, 3.5)
  line L264 (-43.5, 16.5) -> (-58.5, 16.5)
  line L265 (-58.5, 16.5) -> (-58.5, 31.5)
  line L266 (-58.5, 31.5) -> (-43.5, 31.5)
  line L267 (-43.5, 31.5) -> (-43.5, 16.5)
  line L268 (47.8004, -18.6752) -> (38.1586, -7.1845)
  line L269 (38.1586, -7.1845) -> (49.6493, 2.4573)
  line L270 (49.6493, 2.4573) -> (59.2911, -9.0334)
  line L271 (59.2911, -9.0334) -> (47.8004, -18.6752)
  line L272 (60.8232, -7.7478) -> (51.1814, 3.7429)
  line L273 (51.1814, 3.7429) -> (62.672, 13.3847)
  line L274 (62.672, 13.3847) -> (72.3139, 1.894)
  line L275 (72.3139, 1.894) -> (60.8232, -7.7478)
  line L276 (71.2576, -26.4059) -> (80.8994, -37.8965)
  line L277 (80.8994, -37.8965) -> (69.4087, -47.5383)
  line L278 (69.4087, -47.5383) -> (59.7669, -36.0477)
  line L279 (59.7669, -36.0477) -> (71.2576, -26.4059)
  line L280 (103.1942, -42.6863) -> (93.5524, -31.1956)
  line L281 (93.5524, -31.1956) -> (105.043, -21.5538)
  line L282 (105.043, -21.5538) -> (114.6848, -33.0445)
  line L283 (114.6848, -33.0445) -> (103.1942, -42.6863)
  line L284 (-79.5, 15.5) -> (-94.5, 15.5)
  line L285 (-94.5, 15.5) -> (-94.5, 30.5)
  line L286 (-94.5, 30.5) -> (-79.5, 30.5)
  line L287 (-79.5, 30.5) -> (-79.5, 15.5)
  line L288 (66.265, -26.6789) -> (54.7743, -36.3207)
  line L289 (54.7743, -36.3207) -> (45.1325, -24.83)
  line L290 (45.1325, -24.83) -> (56.6232, -15.1882)
  line L291 (56.6232, -15.1882) -> (66.265, -26.6789)
  line L292 (-72.5, 59.5) -> (-72.5, 71.5)
  line L293 (-72.5, 71.5) -> (-90.5, 71.5)
  line L294 (-90.5, 71.5) -> (-90.5, 75.5)
  line L295 (-90.5, 75.5) -> (-119.5, 75.5)
  line L296 (-119.5, 75.5) -> (-119.5, 12.5)
  line L297 (-119.5, 12.5) -> (-101.5, 12.5)
  line L298 (-101.5, 12.5) -> (-101.5, 8.5)
  line L299 (-101.5, 8.5) -> (-83.5, 8.5)
  line L300 (-83.5, 8.5) -> (-83.5, -3.5)
  line L301 (-83.5, -3.5) -> (-65.5, -3.5)
  line L302 (-65.5, -3.5) -> (-65.5, -7.5)
  line L303 (-65.5, -7.5) -> (-36.5, -7.5)
  line L304 (-36.5, -7.5) -> (-36.5, -1.5)
  line L305 (-36.5, -1.5) -> (-18.5, -1.5)
  line L306 (-18.5, -1.5) -> (-18.5, 0.5)
  line L307 (-18.5, 0.5) -> (0.1108, 0.5)
  line L308 (0.1108, 0.5) -> (4.8433, -1.7068)
  line L309 (4.8433, -1.7068) -> (16.8061, -15.9635)
  line L310 (16.8061, -15.9635) -> (15.274, -17.2491)
  line L311 (15.274, -17.2491) -> (26.8442, -31.0379)
  line L312 (26.8442, -31.0379) -> (22.248, -34.8946)
  line L313 (22.248, -34.8946) -> (40.8888, -57.1099)
  line L314 (40.8888, -57.1099) -> (43.953, -54.5388)
  line L315 (43.953, -54.5388) -> (55.5231, -68.3276)
  line L316 (55.5231, -68.3276) -> (64.7157, -60.6141)
  line L317 (64.7157, -60.6141) -> (76.2859, -74.4029)
  line L318 (76.2859, -74.4029) -> (79.35, -71.8318)
  line L319 (79.35, -71.8318) -> (90.9202, -85.6206)
  line L320 (90.9202, -85.6206) -> (139.181, -45.1249)
  line L321 (139.181, -45.1249) -> (120.5402, -22.9096)
  line L322 (120.5402, -22.9096) -> (117.476, -25.4808)
  line L323 (117.476, -25.4808) -> (105.9058, -11.692)
  line L324 (105.9058, -11.692) -> (96.7133, -19.4055)
  line L325 (96.7133, -19.4055) -> (85.1431, -5.6167)
  line L326 (85.1431, -5.6167) -> (82.0789, -8.1878)
  line L327 (82.0789, -8.1878) -> (77.5794, -2.8255)
  line L328 (77.5794, -2.8255) -> (82.1757, 1.0312)
  line L329 (82.1757, 1.0312) -> (77.6762, 6.3935)
  line L330 (77.6762, 6.3935) -> (95.2952, 21.1777)
  line L331 (95.2952, 21.1777) -> (58.4062, 65.1403)
  line L332 (58.4062, 65.1403) -> (16.8892, 84.5)
  line L333 (16.8892, 84.5) -> (-40.5, 84.5)
  line L334 (-40.5, 84.5) -> (-40.5, 61.5)
  line L335 (-40.5, 61.5) -> (-47.5, 61.5)
  line L336 (-47.5, 61.5) -> (-47.5, 55.5)
  line L337 (-47.5, 55.5) -> (-54.5, 55.5)
  line L338 (-54.5, 55.5) -> (-54.5, 59.5)
  line L339 (-54.5, 59.5) -> (-72.5, 59.5)
  line L340 (-7.5, 41.5) -> (-22.5, 41.5)
  line L341 (-22.5, 41.5) -> (-22.5, 56.5)
  line L342 (-22.5, 56.5) -> (-7.5, 56.5)
  line L343 (-7.5, 56.5) -> (-7.5, 41.5)
  line L344 (93.9221, -26.9691) -> (82.4315, -36.611)
  line L345 (82.4315, -36.611) -> (72.7896, -25.1203)
  line L346 (72.7896, -25.1203) -> (84.2803, -15.4785)
  line L347 (84.2803, -15.4785) -> (93.9221, -26.9691)
  line L348 (-97.5, 53.5) -> (-112.5, 53.5)
  line L349 (-112.5, 53.5) -> (-112.5, 68.5)
  line L350 (-112.5, 68.5) -> (-97.5, 68.5)
  line L351 (-97.5, 68.5) -> (-97.5, 53.5)
  line L352 (-61.5, 20.5) -> (-76.5, 20.5)
  line L353 (-76.5, 20.5) -> (-76.5, 35.5)
  line L354 (-76.5, 35.5) -> (-61.5, 35.5)
  line L355 (-61.5, 35.5) -> (-61.5, 20.5)
  line L356 (-43.5, -0.5) -> (-58.5, -0.5)
  line L357 (-58.5, -0.5) -> (-58.5, 14.5)
  line L358 (-58.5, 14.5) -> (-43.5, 14.5)
  line L359 (-43.5, 14.5) -> (-43.5, -0.5)
  line L360 (58.1553, -13.9026) -> (69.646, -4.2608)
  line L361 (69.646, -4.2608) -> (79.2878, -15.7515)
  line L362 (79.2878, -15.7515) -> (67.7971, -25.3933)
  line L363 (67.7971, -25.3933) -> (58.1553, -13.9026)
  line L364 (15.0978, -3.0375) -> (26.5884, 6.6043)
  line L365 (26.5884, 6.6043) -> (36.2303, -4.8864)
  line L366 (36.2303, -4.8864) -> (24.7396, -14.5282)
  line L367 (24.7396, -14.5282) -> (15.0978, -3.0375)
  line L368 (-97.5, 34.5) -> (-97.5, 19.5)
  line L369 (-97.5, 19.5) -> (-112.5, 19.5)
  line L370 (-112.5, 19.5) -> (-112.5, 34.5)
  line L371 (-112.5, 34.5) -> (-97.5, 34.5)
  line L372 (-94.5, 32.5) -> (-94.5, 47.5)
  line L373 (-94.5, 47.5) -> (-79.5, 47.5)
  line L374 (-79.5, 47.5) -> (-79.5, 32.5)
  line L375 (-79.5, 32.5) -> (-94.5, 32.5)
  line L376 (-40.5, 39.5) -> (-40.5, 54.5)
  line L377 (-40.5, 54.5) -> (-25.5, 54.5)
  line L378 (-25.5, 54.5) -> (-25.5, 39.5)
  line L379 (-25.5, 39.5) -> (-40.5, 39.5)
  line L380 (-94.5, 64.5) -> (-79.5, 64.5)
  line L381 (-79.5, 64.5) -> (-79.5, 49.5)
  line L382 (-79.5, 49.5) -> (-94.5, 49.5)
  line L383 (-94.5, 49.5) -> (-94.5, 64.5)
  line L384 (-76.5, 37.5) -> (-76.5, 52.5)
  line L385 (-76.5, 52.5) -> (-61.5, 52.5)
  line L386 (-61.5, 52.5) -> (-61.5, 37.5)
  line L387 (-61.5, 37.5) -> (-76.5, 37.5)
  line L388 (75.7916, 33.5311) -> (85.4334, 22.0405)
  line L389 (85.4334, 22.0405) -> (73.9427, 12.3986)
  line L390 (73.9427, 12.3986) -> (64.3009, 23.8893)
  line L391 (64.3009, 23.8893) -> (75.7916, 33.5311)
  line L392 (62.2758, 16.9684) -> (50.7851, 7.3266)
  line L393 (50.7851, 7.3266) -> (41.1433, 18.8173)
  line L394 (41.1433, 18.8173) -> (52.634, 28.4591)
  line L395 (52.634, 28.4591) -> (62.2758, 16.9684)
  line L396 (-7.5, 7.5) -> (-22.5, 7.5)
  line L397 (-22.5, 7.5) -> (-22.5, 22.5)
  line L398 (-22.5, 22.5) -> (-7.5, 22.5)
  line L399 (-7.5, 22.5) -> (-7.5, 7.5)
  line L400 (67.8766, -48.8239) -> (56.3859, -58.4657)
  line L401 (56.3859, -58.4657) -> (46.7441, -46.9751)
  line L402 (46.7441, -46.9751) -> (58.2348, -37.3333)
  line L403 (58.2348, -37.3333) -> (67.8766, -48.8239)
  line L404 (-18.5, 77.5) -> (-18.5, 62.5)
  line L405 (-18.5, 62.5) -> (-33.5, 62.5)
  line L406 (-33.5, 62.5) -> (-33.5, 77.5)
  line L407 (-33.5, 77.5) -> (-18.5, 77.5)
  line L408 (82.1412, -64.2681) -> (93.6319, -54.6263)
  line L409 (93.6319, -54.6263) -> (103.2737, -66.1169)
  line L410 (103.2737, -66.1169) -> (91.783, -75.7587)